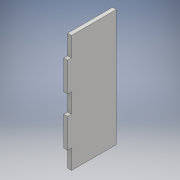
# Autodesk Inventor part: Mounting_wall
Saved by Autodesk Inventor 2017 (Build 210142000, 142)
## iProperties
Created: 2017-11-15
Part Number: Mounting_wall
Material: Generic
Document SubType Name: Modeling
Designer: julie
Density: 1 g/cm^3
Appearance: Default
Author: julie
Autodesk Inventor part; units mm, degrees
ref_plane "YZ Plane" through (0, 0, 0) normal (1, 0, 0) x (0, 1, 0)
ref_plane "XZ Plane" through (0, 0, 0) normal (0, 1, 0) x (-1, 0, 0)
ref_plane "XY Plane" through (0, 0, 0) normal (0, 0, 1) x (1, 0, 0)
sketch "Sketch1" plane through (0, 0, 0) normal (1, 0, 0) x (0, 1, 0)
  line L0 (0, 0) -> (23, 0)
  line L1 (23, 0) -> (23, -60)
  line L2 (23, -60) -> (0, -60)
  line L3 (0, -10) -> (-2, -10)
  line L4 (-2, -10) -> (-2, -25)
  line L5 (-2, -25) -> (0, -25)
  line L6 (0, -50) -> (-2, -50)
  line L7 (-2, -50) -> (-2, -35)
  line L8 (-2, -35) -> (0, -35)
  line L9 (0, -10) -> (0, 0)
  line L10 (0, -60) -> (0, -50)
  line L11 (0, -35) -> (0, -25)
  dimension "d0" = 23
  dimension "d1" = 60
  dimension "d2" = 2
  dimension "d3" = 15
  dimension "d4" = 10
  dimension "d5" = 15
  dimension "d6" = 10
  dimension "d10" = 2
  dimension "d11" = 0
  dimension "d12" = 2
  constraints: 24 end point, 9 perpendicular, 4 parallel, 3 horizontal
  measures "d0" distance of L1.end L2.end
  measures "d1" distance of L0.end L1.end
  measures "d2" distance of L3.start L3.end
  measures "d3" distance of L3.end L4.end
  measures "d4" distance from line of L0.start L3
  measures "d5" distance of L6.end L7.end
  measures "d6" distance between parallel lines of L2 L6
  measures "d10" distance of L6.start L6.end
  measures "d11" distance from line of L0.start L11
  measures "d12" distance of L7.end L8.end
extrude "Extrusion1" add sketch "Sketch1" along normal blind 2
body "Solid1"
